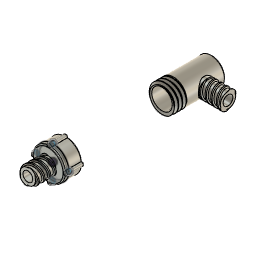
chamber top and bottom (1) (Autodesk Fusion 360 design; units mm, degrees)
Autodesk Fusion 360 part; units mm, degrees
sketch "Sketch1" plane through (0, 0, 0) normal (0, 1, 0) x (1, 0, 0)
  circle A0 centre (0, 0) radius 6
  circle A1 centre (0, 0) radius 4.5
  dimension "d1" = 12
  dimension "d2" = 9
  constraint coincident A0.centre A1.centre
  measures "d1" diameter of A0
  measures "d2" diameter of A1
extrude "Extrude1" add sketch "Sketch1" along normal blind 22 contours A0 | A1 makes body 1
extrude "Extrude2" cut sketch "Sketch1" along normal blind 22 contours A1 bodies 1
thread "Thread1" "ISO Metric profile 12.0 M12x1.75 6g" major diameter 11.8335 minor diameter 9.8365 pitch 1.75 angle 60 modelled right hand crest width 0.2518 on face at (5.9925, 14.6667, 0.2991) from (0, 0, 0) to (0, 5, 0) crest through (5.9168, -0.4375, 0) on bodies 1
sketch "Sketch2" plane through (0, 0, 0) normal (1, 0, 0) x (0, 1, 0)
  circle A0 through (17.9, 0, 6) (12.05, 3.3775, 6) (12.05, -3.3775, 6)
  circle A1 through (16.15, 0, 6) (12.925, 1.862, 6) (12.925, -1.862, 6)
  circle A2 through (15.88, 0, 6) (13.06, 1.6281, 6) (13.06, -1.6281, 6)
  dimension "d9" = 7.8
  dimension "d10" = 4.3
  dimension "d11" = 3.76
extrude "Extrude7" add sketch "Sketch2" against normal blind 1.5 contours A0 | A1 | A2 in plane through (6, 0, 0) normal (1, 0, 0) bodies 1
sketch "Sketch4" plane through (6, 0, 0) normal (1, 0, 0) x (0, 1, 0)
  circle A0 centre (14, 0) radius 3.35
  circle A1 centre (14, 0) radius 1.8795
  arc A2 (12.76, 3.695) -> (10.5928, 1.8925) centre (14, 0) ccw
  arc A3 (14.004, 3.3446) -> (12.76, 3.695) centre (12.513, 0.435) ccw
  arc A4 (10.5928, 1.8925) -> (10.7079, 0.6045) centre (13.844, 1.534) ccw
  arc A5 (15.24, -3.695) -> (17.4072, -1.8925) centre (14, 0) ccw
  arc A6 (13.996, -3.3446) -> (15.24, -3.695) centre (15.487, -0.435) ccw
  arc A7 (17.4072, -1.8925) -> (17.2921, -0.6045) centre (14.156, -1.534) ccw
  line L0 (14, 0, 0) -> (14, 0, 9)
extrude "Extrude8" add sketch "Sketch4" along normal blind 9 contours A0 bodies 1
extrude "Extrude9" cut sketch "Sketch4" along normal blind 9 draft 1.72 contours A1 bodies 1
sweep "Sweep2" add twist angle 648 profiles "Sketch4" path "Sketch4" along L0 section 1 contours A0 A2 A3 A4 | A0 A5 A6 A7 bodies 1
extrude "Extrude10" cut sketch "Sketch2" against normal blind 2 contours A2 in plane through (6, 0, 0) normal (1, 0, 0) bodies 1
move_body "Move1" bodies 1 to x (1, 0, 0) y (0, 1, 0) z (0, 0, 1) at (0, 48, 0)
sketch "Sketch5" plane through (0, 0, 0) normal (0, 1, 0) x (1, 0, 0)
  circle A0 centre (0, 0) radius 6.05
  circle A1 centre (0, 0) radius 7
  circle A2 centre (7, 0) radius 0.9
  circle A3 centre (-7, 0) radius 0.9
  circle A4 centre (0, 7) radius 0.9
  circle A5 centre (0, -7) radius 0.9
  dimension "d40" = 12.1
  dimension "d41" = 14
  constraint coincident A0.centre A1.centre
  constraint concentric A0 A1
  constraint coincident A1 A2.centre
  constraint coincident A1 A3.centre
  constraint coincident A1 A4.centre
  constraint coincident A1 A5.centre
  measures "d40" diameter of A0
  measures "d41" diameter of A1
extrude "Extrude11" add sketch "Sketch5" along normal blind 6 separate body contours A1 A2 | A1 A2 A3 A4 A5 | A1 A4 | A1 A5 | A1 A3 picked at (6.7169, 0.2054) picked at (0.0215, 6.6965) picked at (-0.0215, -6.6965) picked at (-6.6957, 0) makes body 2
thread "Thread2" "ISO Metric profile 12.0 M12x1.75 6H" major diameter 12.2265 minor diameter 10.2735 pitch 1.75 angle 60 modelled right hand crest width 0.4769 on face at (6.0425, 4, 0.3016) crest through (5.1368, 0.4375, 0) on bodies 2
extrude "Extrude12" add sketch "Sketch5" against normal blind 2 contours A0 | A1 A2 | A1 A2 A3 A4 A5 | A1 A4 | A1 A5 | A1 A3 picked at (6.7169, 0.2054) picked at (0.0215, 6.6965) picked at (-0.0215, -6.6965) picked at (-6.6957, 0) bodies 2
sketch "Sketch6" plane through (0, -2, 0) normal (0, -1, 0) x (-1, 0, 0)
  circle A0 centre (0, 0) radius 3.35
  circle A1 centre (0, 0) radius 1.8795
  arc A2 (-1.24, 3.695) -> (-3.4072, 1.8925) centre (0, 0) ccw
  arc A3 (0.004, 3.3446) -> (-1.24, 3.695) centre (-1.487, 0.435) ccw
  arc A4 (-3.4072, 1.8925) -> (-3.2921, 0.6045) centre (-0.156, 1.534) ccw
  arc A5 (1.24, -3.695) -> (3.4072, -1.8925) centre (0, 0) ccw
  arc A6 (-0.004, -3.3446) -> (1.24, -3.695) centre (1.487, -0.435) ccw
  arc A7 (3.4072, -1.8925) -> (3.2921, -0.6045) centre (0.156, -1.534) ccw
  line L0 (0, 0, 0) -> (0, 0, 9)
extrude "Extrude13" add sketch "Sketch6" along normal blind 9 contours A0 bodies 2
extrude "Extrude14" cut sketch "Sketch6" along normal blind 9 draft 1.72 contours A1 bodies 2
sweep "Sweep3" add twist angle 648 profiles "Sketch6" path "Sketch6" along L0 section 1 contours A0 A2 A3 A4 | A0 A5 A6 A7 bodies 2
extrude "Extrude15" cut 1 faces at (0.5681, -2, -0.0732) along direction (0, 1, 0) blind 2 on bodies 2 bodies 2
extrude "Extrude16" add sketch "Sketch5" along normal blind 6 and the other way blind 2 contours A1 A2 | A1 A4 | A1 A5 | A1 A3 picked at (7.2847, 0.1879) picked at (-0.0096, 7.2956) picked at (-0.0096, -7.2956) picked at (-7.2957, 0) bodies 2
fillet "Fillet1" radius 0.5 8 edges at (-4.9497, 6, 4.9497) (4.9497, 6, 4.9497) (4.9497, 6, -4.9497) (-4.9497, 6, -4.9497) (0, 6, -7.9) (-7.9, 6, 0) (0, 6, 7.9) (7.9, 6, 0) on bodies 2
fillet "Fillet2" radius 0.5 1 edges at (-5.5163, 70, 2.1396) on bodies 1
fillet "Fillet3" radius 0.5 7 edges at (4.9497, -2, -4.9497) (4.9497, -2, 4.9497) (-4.9497, -2, 4.9497) (-4.9497, -2, -4.9497) (-7.9, -2, 0) (0, -2, 7.9) (7.9, -2, 0) on bodies 2
fillet "Fillet4" radius 0.5 1 edges at (0, -2, -7.9) on bodies 2
extrude "Extrude3" [suppressed]
sketch "Sketch3" plane through (6, 0, 0) normal (1, 0, 0) x (0, 1, 0)
  circle A0 centre (12, 0) radius 3.35
  circle A1 centre (12, 0) radius 1.8795
  arc A2 (10.76, 3.695) -> (8.5928, 1.8925) centre (12, 0) ccw
  arc A3 (12.004, 3.3446) -> (10.76, 3.695) centre (10.513, 0.435) ccw
  arc A4 (8.5928, 1.8925) -> (8.7079, 0.6045) centre (11.844, 1.534) ccw
  arc A5 (13.24, -3.695) -> (15.4072, -1.8925) centre (12, 0) ccw
  arc A6 (11.996, -3.3446) -> (13.24, -3.695) centre (13.487, -0.435) ccw
  arc A7 (15.4072, -1.8925) -> (15.2921, -0.6045) centre (12.156, -1.534) ccw
  line L0 (12, 0, 0) -> (12, 0, 9)
extrude "Extrude4" [suppressed]
extrude "Extrude5" [suppressed]
sweep "Sweep1" [suppressed]
extrude "Extrude6" [suppressed]
